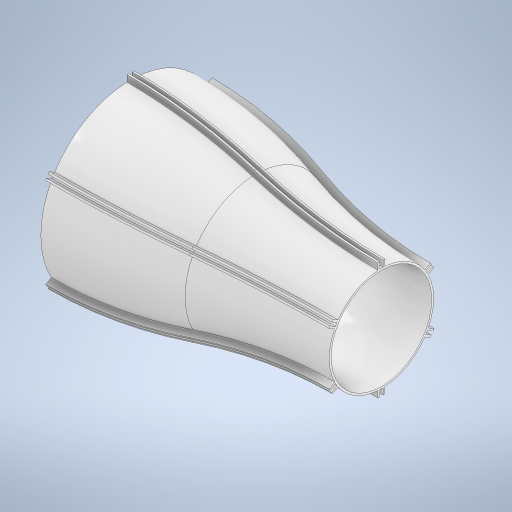
# Autodesk Inventor part: Düse
Saved by Autodesk Inventor 2023 (Build 270158000, 158)
## iProperties
Created: 2022-02-27
Part Number: Düse
Material: Generisch
Document SubType Name: Modeling
Designer: Marcel
Density: 1 g/cm^3
Appearance: Weiß
Author: Marcel
Autodesk Inventor part; units mm, degrees
ref_plane "YZ Plane" through (0, 0, 0) normal (1, 0, 0) x (0, 1, 0)
ref_plane "XZ Plane" through (0, 0, 0) normal (0, 1, 0) x (-1, 0, 0)
ref_plane "XY Plane" through (0, 0, 0) normal (0, 0, 1) x (1, 0, 0)
sketch "Skizze9" plane through (0, 0, 0) normal (0, 0, 1) x (1, 0, 0)
  line L0 (0, 0) -> (200, 0)
  line L1 (200, 0) -> (200, 40.1)
  line L2 (200, 40.1) -> (200, 41.6)
  line L3 (0, 0) -> (0, 70)
  line L4 (0, 70) -> (0, 71.5)
  arc A0 (100, 55.05) -> (0, 70) centre (0, -271.9232) ccw
  arc A1 (100, 55.05) -> (200, 40.1) centre (200, 382.0232) ccw
  arc A2 (100, 56.55) -> (0, 71.5) centre (0, -270.4232) ccw
  arc A3 (100, 56.55) -> (200, 41.6) centre (200, 383.5232) ccw
  line L5 (0, 71.5) -> (0, 101.5)
  line L6 (200, 41.6) -> (200, 78.6)
  line L7 (0, 101.5) -> (0, 103)
  line L8 (200, 78.6) -> (200, 80.1)
  line L9 (0, 103) -> (0, 133)
  line L10 (0, 133) -> (0, 134.5)
  line L11 (200, 80.1) -> (200, 122.4)
  line L12 (200, 122.4) -> (200, 123.9)
  arc A4 (100, 90.05) -> (200, 78.6) centre (200, 521.0062) ccw
  arc A5 (100, 91.55) -> (200, 80.1) centre (200, 522.5062) ccw
  arc A6 (100, 90.05) -> (0, 101.5) centre (0, -340.9062) ccw
  arc A7 (100, 91.55) -> (0, 103) centre (0, -339.4062) ccw
  arc A8 (100, 129.2) -> (200, 123.9) centre (200, 1069.9462) ccw
  arc A9 (100, 127.7) -> (0, 133) centre (0, -813.0462) ccw
  arc A10 (100, 127.7) -> (200, 122.4) centre (200, 1068.4462) ccw
  arc A11 (100, 129.2) -> (0, 134.5) centre (0, -811.5462) ccw
  arc A12 (101.4623, 61.3314) -> (0, 76.5) centre (0, -270.4232) ccw
  arc A13 (101.4623, 61.3314) -> (200, 46.6) centre (200, 383.5232) ccw
  point P0 (143.9749, 47.5506)
  point P1 (136.2206, 124.2462)
  point P2 (104.2284, 54.3303)
  point P3 (200, 46.6)
  point P4 (0, 76.5)
  point P5 (200, 46.6)
  point P6 (0, 76.5)
  dimension "d103" = 200
  dimension "d104" = 40.1
  dimension "d105" = 1.5
  dimension "d106" = 70
  dimension "d107" = 1.5
  dimension "d108" = 30
  dimension "d109" = 37
  dimension "d110" = 1.5
  dimension "d111" = 1.5
  dimension "d112" = 30
  dimension "d113" = 1.5
  dimension "d114" = 42.3
  dimension "d115" = 1.5
  dimension "d116" = 100
  dimension "d117" = 100
  dimension "d118" = 100
  dimension "d119" = 5
  constraints: 28 point on circle, 26 end point, 14 centre point, 9 equal radius, 9 line through centre, 7 vertical, 4 point on line, 4 vertical alignment, 1 coincident, 1 horizontal, 1 perpendicular, 1 other
  measures "d103" distance of L0.start L0.end
  measures "d104" distance of L0.end L1.end
  measures "d105" distance of L1.end L2.end
  measures "d106" distance of L0.start L3.end
  measures "d107" distance of L3.end L4.end
  measures "d108" distance of L4.end L5.end
  measures "d109" distance of L2.end L6.end
  measures "d110" distance of L5.end L7.end
  measures "d111" distance of L6.end L8.end
  measures "d112" distance of L7.end L9.end
  measures "d113" distance of L9.end L10.end
  measures "d114" distance of L8.end L11.end
  measures "d115" distance of L11.end L12.end
  measures "d116" distance from line of L3 A0.start
  measures "d117" distance from line of L5 A4.start
  measures "d118" distance from line of L9 A9.start
  measures "d119" radial gap between concentric circles of A2 A12
sketch "Skizze10" plane through (0, 0, 0) normal (0, 0, 1) x (1, 0, 0)
  line L0 (0, 0) -> (200, 0)
  line L1 (200, 0) -> (200, 40.1)
  line L2 (200, 40.1) -> (200, 41.6)
  line L3 (0, 0) -> (0, 70)
  line L4 (0, 70) -> (0, 71.5)
  arc A0 (100, 55.05) -> (0, 70) centre (0, -271.9232) ccw
  arc A1 (100, 55.05) -> (200, 40.1) centre (200, 382.0232) ccw
  line L5 (0, 71.5) -> (0, 101.5)
  line L6 (200, 41.6) -> (200, 78.6)
  line L7 (0, 101.5) -> (0, 103)
  line L8 (200, 78.6) -> (200, 80.1)
  line L9 (0, 103) -> (0, 133)
  line L10 (0, 133) -> (0, 134.5)
  line L11 (200, 80.1) -> (200, 122.4)
  line L12 (200, 122.4) -> (200, 123.9)
  arc A2 (100, 90.05) -> (200, 78.6) centre (200, 521.0062) ccw
  arc A3 (100, 91.55) -> (200, 80.1) centre (200, 522.5062) ccw
  arc A4 (100, 90.05) -> (0, 101.5) centre (0, -340.9062) ccw
  arc A5 (100, 91.55) -> (0, 103) centre (0, -339.4062) ccw
  arc A6 (100, 129.2) -> (200, 123.9) centre (200, 1069.9462) ccw
  arc A7 (100, 127.7) -> (0, 133) centre (0, -813.0462) ccw
  arc A8 (100, 127.7) -> (200, 122.4) centre (200, 1068.4462) ccw
  arc A9 (100, 129.2) -> (0, 134.5) centre (0, -811.5462) ccw
  arc A10 (101.4623, 61.3314) -> (0, 76.5) centre (0, -270.4232) ccw
  arc A11 (101.4623, 61.3314) -> (200, 46.6) centre (200, 383.5232) ccw
  point P0 (143.9749, 47.5506)
  point P1 (136.2206, 124.2462)
  point P2 (104.2284, 54.3303)
  point P3 (200, 46.6)
  point P4 (0, 76.5)
  point P5 (200, 46.6)
  point P6 (0, 76.5)
  point P7 (200, 46.6)
  point P8 (0, 76.5)
  point P9 (200, 46.6)
  point P10 (0, 76.5)
  dimension "d120" = 200
  dimension "d121" = 40.1
  dimension "d122" = 1.5
  dimension "d123" = 70
  dimension "d124" = 1.5
  dimension "d125" = 30
  dimension "d126" = 37
  dimension "d127" = 1.5
  dimension "d128" = 1.5
  dimension "d129" = 30
  dimension "d130" = 1.5
  dimension "d131" = 42.3
  dimension "d132" = 1.5
  dimension "d133" = 100
  dimension "d134" = 100
  dimension "d135" = 100
  constraints: 26 end point, 24 point on circle, 12 centre point, 7 line through centre, 7 vertical, 6 equal radius, 4 point on line, 3 vertical alignment, 1 coincident, 1 horizontal, 1 perpendicular
  measures "d120" distance of L0.start L0.end
  measures "d121" distance of L0.end L1.end
  measures "d122" distance of L1.end L2.end
  measures "d123" distance of L0.start L3.end
  measures "d124" distance of L3.end L4.end
  measures "d125" distance of L4.end L5.end
  measures "d126" distance of L2.end L6.end
  measures "d127" distance of L5.end L7.end
  measures "d128" distance of L6.end L8.end
  measures "d129" distance of L7.end L9.end
  measures "d130" distance of L9.end L10.end
  measures "d131" distance of L8.end L11.end
  measures "d132" distance of L11.end L12.end
  measures "d133" distance from line of L3 A0.start
  measures "d134" distance from line of L5 A2.start
  measures "d135" distance from line of L9 A7.start
revolve "Umdrehung4" add sketch "Skizze9" angle 360 about axis through (0, 0, 0) along (1, 0, 0) contours L4 A2 A3 L2 A1 A0
extrude "Extrusion4" add sketch "Skizze10" along normal mid plane 5.5 contours L4 L5 A10 A11 L6 L2 A1 A0
sketch "Skizze12" plane through (0, 0, 0) normal (0, 0, 1) x (1, 0, 0)
  line L0 (0, 0) -> (200, 0)
  line L1 (200, 0) -> (200, 40.1)
  line L2 (200, 40.1) -> (200, 41.6)
  line L3 (0, 0) -> (0, 70)
  line L4 (0, 70) -> (0, 71.5)
  arc A0 (100, 55.05) -> (0, 70) centre (0, -271.9232) ccw
  arc A1 (100, 55.05) -> (200, 40.1) centre (200, 382.0232) ccw
  arc A2 (100, 56.55) -> (0, 71.5) centre (0, -270.4232) ccw
  arc A3 (100, 56.55) -> (200, 41.6) centre (200, 383.5232) ccw
  line L5 (0, 71.5) -> (0, 101.5)
  line L6 (200, 41.6) -> (200, 78.6)
  line L7 (0, 101.5) -> (0, 103)
  line L8 (200, 78.6) -> (200, 80.1)
  line L9 (0, 103) -> (0, 133)
  line L10 (0, 133) -> (0, 134.5)
  line L11 (200, 80.1) -> (200, 122.4)
  line L12 (200, 122.4) -> (200, 123.9)
  arc A4 (100, 90.05) -> (200, 78.6) centre (200, 521.0062) ccw
  arc A5 (100, 91.55) -> (200, 80.1) centre (200, 522.5062) ccw
  arc A6 (100, 90.05) -> (0, 101.5) centre (0, -340.9062) ccw
  arc A7 (100, 91.55) -> (0, 103) centre (0, -339.4062) ccw
  arc A8 (100, 129.2) -> (200, 123.9) centre (200, 1069.9462) ccw
  arc A9 (100, 127.7) -> (0, 133) centre (0, -813.0462) ccw
  arc A10 (100, 127.7) -> (200, 122.4) centre (200, 1068.4462) ccw
  arc A11 (100, 129.2) -> (0, 134.5) centre (0, -811.5462) ccw
  arc A12 (101.4623, 61.3314) -> (0, 76.5) centre (0, -270.4232) ccw
  arc A13 (101.4623, 61.3314) -> (200, 46.6) centre (200, 383.5232) ccw
  point P0 (143.9749, 47.5506)
  point P1 (136.2206, 124.2462)
  point P2 (104.2284, 54.3303)
  point P3 (200, 46.6)
  point P4 (0, 76.5)
  point P5 (200, 46.6)
  point P6 (0, 76.5)
  point P7 (200, 46.6)
  point P8 (0, 76.5)
  dimension "d142" = 200
  dimension "d143" = 40.1
  dimension "d144" = 1.5
  dimension "d145" = 70
  dimension "d146" = 1.5
  dimension "d147" = 30
  dimension "d148" = 37
  dimension "d149" = 1.5
  dimension "d150" = 1.5
  dimension "d151" = 30
  dimension "d152" = 1.5
  dimension "d153" = 42.3
  dimension "d154" = 1.5
  dimension "d155" = 100
  dimension "d156" = 100
  dimension "d157" = 100
  dimension "d158" = 5
  constraints: 28 point on circle, 26 end point, 14 centre point, 9 equal radius, 9 line through centre, 7 vertical, 4 point on line, 4 vertical alignment, 1 coincident, 1 horizontal, 1 perpendicular, 1 other
  measures "d142" distance of L0.start L0.end
  measures "d143" distance of L0.end L1.end
  measures "d144" distance of L1.end L2.end
  measures "d145" distance of L0.start L3.end
  measures "d146" distance of L3.end L4.end
  measures "d147" distance of L4.end L5.end
  measures "d148" distance of L2.end L6.end
  measures "d149" distance of L5.end L7.end
  measures "d150" distance of L6.end L8.end
  measures "d151" distance of L7.end L9.end
  measures "d152" distance of L9.end L10.end
  measures "d153" distance of L8.end L11.end
  measures "d154" distance of L11.end L12.end
  measures "d155" distance from line of L3 A0.start
  measures "d156" distance from line of L5 A4.start
  measures "d157" distance from line of L9 A9.start
  measures "d158" radial gap between concentric circles of A2 A12
extrude "Extrusion5" cut sketch "Skizze12" along normal mid plane 2.5 contours L5 A12 A13 L6 A3 A2
pattern_circular "Runde Anordnung4" count 6 over 360 about axis through (-10, 0, 0) along (1, 0, 0) of "Extrusion4", "Extrusion5"
